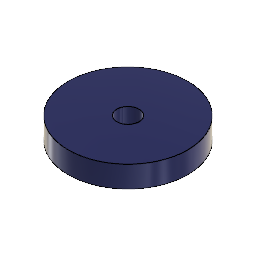
2-Roller_Insert v1 v3 (Autodesk Fusion 360 design; units mm, degrees)
Autodesk Fusion 360 part; units mm, degrees
sketch "Roller_Insert" plane through (0, 0, 0) normal (0, 0, 1) x (1, 0, 0)
  circle A0 centre (0, 0) radius 34.925
  dimension "d1" = 69.85
  constraint coincident A0.centre origin
  measures "d1" diameter of A0
extrude "Extrude2" add sketch "Roller_Insert" along normal blind 12.7
sketch "Pipe Cutout" plane through (0, 0, 12.7) normal (0, 0, 1) x (-1, 0, 0)
  circle A0 centre (0, 0) radius 34.925
  circle A1 centre (0, 0) radius 6.45
  dimension "d9" = 12.9
  constraint concentric A0 A1
  measures "d9" diameter of A1
extrude "Extrude3" cut sketch "Pipe Cutout" against normal through all contours A1
named bodies: "Roller Insert"
